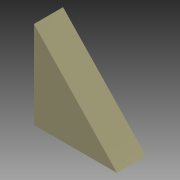
# Autodesk Inventor part: nylon thing
Saved by Autodesk Inventor 2013 (Build 170138000, 138)
## iProperties
Created: 2013-02-04
Part Number: nylon thing
Material: Nylon 6/6
Document SubType Name: Modeling
Designer: Arpan
Density: 1 g/cm^3
Author: Arpan
Autodesk Inventor part; units mm, degrees
ref_plane "YZ Plane" through (0, 0, 0) normal (1, 0, 0) x (0, 1, 0)
ref_plane "XZ Plane" through (0, 0, 0) normal (0, 1, 0) x (-1, 0, 0)
ref_plane "XY Plane" through (0, 0, 0) normal (0, 0, 1) x (1, 0, 0)
sketch "Sketch1" plane through (0, 0, 0) normal (0, 0, 1) x (1, 0, 0)
  line L0 (0, 0) -> (-72.39, 0)
  line L1 (-72.39, 0) -> (-72.39, 76.2)
  line L2 (-72.39, 76.2) -> (0, 0)
  dimension "d0" = 72.39
  dimension "d1" = 76.2
  dimension "d2" = 90
  constraints: 6 end point, 1 horizontal
  measures "d0" distance of L0.start L0.end
  measures "d1" distance of L0.end L1.end
  measures "d2" angle of L0 L1
extrude "Extrusion1" add sketch "Sketch1" along normal blind 25.4
body "Solid1"
